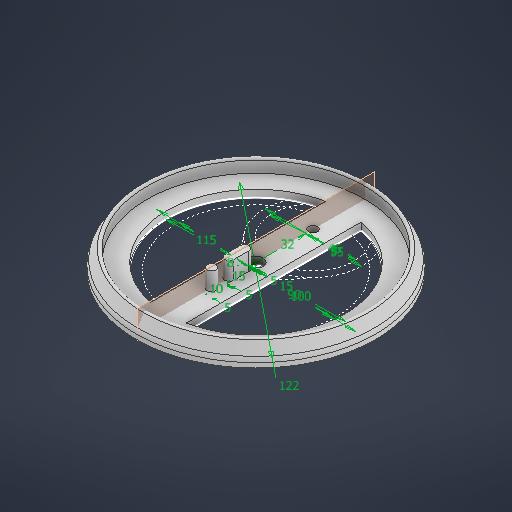
# Autodesk Inventor part: Gear Holder 2
Saved by Autodesk Inventor 2026.2 (Build 302298000, 298)
## iProperties
Created: 2026-01-26
Part Number: Gear Holder 2
Material: Generic
Document SubType Name: Modeling
Designer: Cobble
Density: 1 g/cm^3
Appearance: Default
Author: Cobble
Autodesk Inventor part; units mm, degrees
ref_plane "YZ Plane" through (0, 0, 0) normal (1, 0, 0) x (0, 1, 0)
ref_plane "XZ Plane" through (0, 0, 0) normal (0, 1, 0) x (-1, 0, 0)
ref_plane "XY Plane" through (0, 0, 0) normal (0, 0, 1) x (1, 0, 0)
sketch "Sketch1" plane through (0, 0, 0) normal (0, 0, 1) x (1, 0, 0)
  circle A0 centre (0, 0) radius 61
  arc A1 (7.0788, 15.7662) -> (7.8803, 16.1398) centre (0, 32) ccw
  circle A2 centre (0, 0) radius 61
  circle A3 centre (0, 32) radius 2.5
  circle A4 centre (0, 0) radius 50
  circle A5 centre (0, 0) radius 57.5 construction
  circle A6 centre (0, 0) radius 57 construction
  circle A7 centre (0, 0) radius 7.5 construction
  circle A8 centre (0, 32) radius 23 construction
  circle A9 centre (0, 0) radius 45 construction
  circle A10 centre (0, 32) radius 27.5 construction
  line L0 (-5.8547, -4.6875) -> (-21.4672, 14.8125) construction
  line L1 (5.8547, -4.6875) -> (21.4672, 14.8125) construction
  line L2 (0, 0) -> (0, 32) construction
  line L3 (7.5, 44.3706) -> (7.5, -44.3706) construction
  line L4 (-7.5, 44.3706) -> (-7.5, -44.3706) construction
  circle A11 centre (0, 0) radius 2.5
  line L5 (0, 0) -> (0, -15) construction
  circle A12 centre (0, -15) radius 2.5
  line L6 (-2.5, 0) -> (-2.5, -15)
  line L7 (2.5, -15) -> (2.5, 0)
  circle A13 centre (0, -7.5) radius 10 construction
  line L8 (-10, -7.5) -> (-10, 60.1747)
  line L9 (10, -7.5) -> (10, 60.1747)
  line L10 (-10, -7.5) -> (-10, -60.1747)
  line L11 (10, -7.5) -> (10, -60.1747)
  circle A14 centre (0, 0) radius 4
  circle A15 centre (0, -6.5) radius 2.5
  line L12 (0, -15) -> (0, -25)
  circle A16 centre (0, -25) radius 2.5
  point P0 (35.0374, 41.2549)
  point P1 (15.3046, 2.7982)
  point P2 (-19.4282, 41.2549)
  point P3 (0.3046, 2.7982)
  point P4 (25.4129, 52.2276)
  point P5 (-9.8037, 52.2276)
  point P6 (-10, 48.9898)
  point P7 (-10, -48.9898)
  point P8 (10, 48.9898)
  point P9 (10, -48.9898)
  point P10 (-2.5, -6.5)
  point P11 (2.5, -6.5)
  point P12 (-2.5, -3.1225)
  point P13 (2.5, -3.1225)
  dimension "d0" = 5
  dimension "d1" = 100
  dimension "d2" = 115
  dimension "d3" = 15
  dimension "d4" = 46
  dimension "d5" = 90
  dimension "d6" = 55
  dimension "d7" = 32
  dimension "d8" = 5
  dimension "d9" = 15
  dimension "d10" = 5
  dimension "d23" = 122
  dimension "d26" = 8
  dimension "d28" = 10
  dimension "d29" = 5
  constraints: 26 end point, 20 point on circle, 17 centre point, 15 coincident, 15 tangent, 6 vertical, 3 parallel, 1 concentric, 1 midpoint, 1 point on line
  measures "d0" diameter of A3
  measures "d1" diameter of A4
  measures "d2" diameter of A5
  measures "d3" diameter of A7
  measures "d4" diameter of A8
  measures "d5" diameter of A9
  measures "d6" diameter of A10
  measures "d7" distance of A1.centre A0.centre
  measures "d8" diameter of A11
  measures "d9" distance of L5.start L5.end
  measures "d10" diameter of A12
  measures "d23" diameter of A2
  measures "d26" diameter of A14
  measures "d28" distance of L12.start L12.end
  measures "d29" diameter of A16
extrude "Extrusion1" add sketch "Sketch1" along normal blind 4 contours A0 L11 A4 L9 | L9 A4 L8 A0 | A0 L10 A4 L11 | L8 A4 L10 A0 | L9 L11 A4 L10 L8 | A16 | L7 A15 A14 | A14 A15 L6 | A15 | L7 A12 L6 A15 | A12
extrude "Extrusion2" add sketch "Sketch1" along normal blind 14 contours A16 | A15 | L7 A12 L6 A15 | A12
ref_plane "Work Plane1" through (0, -48.9898, 0) normal (1, 0, 0) x (0, 0, -1)
sketch "Sketch2" plane through (0, -48.9898, 0) normal (1, 0, 0) x (0, 0, -1)
  line L0 (-4, 109.9898) -> (-4, -12.0102) projected
  line L1 (0, 109.9898) -> (0, -12.0102) projected
  line L2 (0, 109.9898) -> (0, -12.0102) projected
  line L3 (0, -12.0102) -> (-10.3897, -12.0102)
  line L4 (-14, 33.9898) -> (-14, 31.4898) projected
  line L5 (0, -12.0102) -> (-4, -12.0102)
  line L6 (-4, -12.0102) -> (-4, -18.0102)
  line L7 (-2.6151, -18.0102) -> (0, -18.0102)
  line L8 (0, -18.0102) -> (0, -12.0102)
  line L9 (-5.1876, -17.2977) -> (-10.9042, -13.8677)
  arc A0 (-10.3897, -12.0102) -> (-10.9042, -13.8677) centre (-10.3897, -13.0102) ccw
  arc A1 (-5.1876, -17.2977) -> (-2.6151, -18.0102) centre (-2.6151, -13.0102) ccw
  line L10 (-0.0174, 48.9898) -> (-14.0174, 48.9898) construction
  line L11 (-0.0174, 48.9898) -> (13.9826, 48.9898) construction
  point P0 (0, 48.9898)
  point P1 (-14, -12.0102)
  dimension "d15" = 14
  dimension "d16" = 4
  dimension "d17" = 6
  dimension "d18" = 1
  dimension "d19" = 5
  dimension "d20" = 14
  dimension "d21" = 180
  constraints: 16 end point, 4 point on circle, 4 point on line, 4 tangent, 3 horizontal, 2 centre point, 2 parallel, 2 perpendicular, 1 collinear
  measures "d15" distance of L1.end point (-14, -12.01)
  measures "d16" distance of L7.end L6.end
  measures "d17" distance of L6.end L5.end
  measures "d18" radius of A0
  measures "d19" radius of A1
  measures "d20" distance of L10.start L10.end
  measures "d21" angle of L10 L11
revolve "Revolution1" add sketch "Sketch2" angle 360 about axis through (0, 0, 0.0174) along (0, 0, 1)
body "Solid1"
